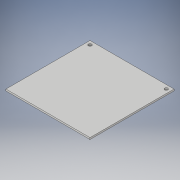
# Autodesk Inventor part: teensy_box_lid
Saved by Autodesk Inventor 2017 (Build 210142000, 142)
## iProperties
Created: 2016-09-21
Part Number: teensy_box_lid
Material: Generic
Document SubType Name: Modeling
Designer: corvera
Density: 1 g/cm^3
Appearance: Default
Author: corvera
Autodesk Inventor part; units mm, degrees
ref_plane "YZ Plane" through (0, 0, 0) normal (1, 0, 0) x (0, 1, 0)
ref_plane "XZ Plane" through (0, 0, 0) normal (0, 1, 0) x (-1, 0, 0)
ref_plane "XY Plane" through (0, 0, 0) normal (0, 0, 1) x (1, 0, 0)
sketch "Sketch1" plane through (0, 0, 0) normal (0, 1, 0) x (-1, 0, 0)
  line L0 (38, 38) -> (-38, 38)
  line L1 (-38, 38) -> (-38, -38)
  line L2 (-38, -38) -> (38, -38)
  line L3 (38, -38) -> (38, 38)
  line L4 (38, 38) -> (-38, -38) construction
  line L5 (-38, 38) -> (38, -38) construction
  point P0 (0, 0)
  dimension "d0" = 76
  dimension "d1" = 76
  constraints: 12 end point, 2 midpoint, 2 parallel, 1 horizontal, 1 perpendicular
  measures "d0" distance of L1.end L2.end
  measures "d1" distance of L0.end L1.end
extrude "Extrusion1" add sketch "Sketch1" along normal blind 1.5
sketch "Sketch2" plane through (0, 0, 0) normal (0, 1, 0) x (-1, 0, 0)
  circle A0 centre (-34.5, -34.5) radius 1.45
  line L0 (-34.5, -34.5) -> (-38, -34.5) construction
  line L1 (-38, 38) -> (-38, -38) construction
  line L2 (-34.5, -34.5) -> (-34.5, -38) construction
  line L3 (-38, -38) -> (38, -38) construction
  line L4 (0, 0) -> (0, -38) construction
  line L5 (-38, -38) -> (38, -38) construction
  circle A1 centre (34.5, -34.5) radius 1.45
  line L6 (34.5, -34.5) -> (38, -34.5) construction
  line L7 (34.5, -34.5) -> (34.5, -38) construction
  dimension "d4" = 2.9
  dimension "d5" = 3.5
  dimension "d6" = 3.5
  constraints: 10 end point, 3 symmetric about line, 2 centre point, 2 point on line, 1 horizontal, 1 midpoint, 1 vertical, 1 other
  measures "d4" diameter of A0
  measures "d5" distance of L0.start L0.end
  measures "d6" distance of L0.start L2.end
extrude "Extrusion2" cut sketch "Sketch2" along normal blind 1.5
body "Solid1"
